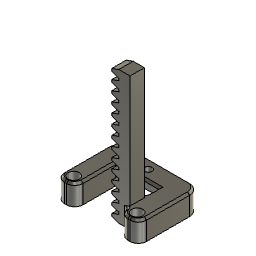
z lifter v18 (Autodesk Fusion 360 design; units mm, degrees)
Autodesk Fusion 360 part; units mm, degrees
note: some values were not read from the file. Chosen so that the rebuilt part matches the saved one: which pieces of a blend or face edit are solid.
sketch "Sketch1" plane through (0, 0, 0) normal (0, 1, 0) x (1, 0, 0)
  line L0 (20, -5) -> (-20, -5)
  line L1 (-20, -5) -> (-20, 5)
  line L2 (-20, 5) -> (20, 5)
  line L3 (20, 5) -> (20, -5)
  line L4 (20, -5) -> (-20, 5) construction
  line L5 (-20, -5) -> (20, 5) construction
  dimension "d1" = 40
  dimension "d2" = 10
  constraint horizontal L0
  constraint perpendicular L0 L1
  constraint parallel L0 L2
  constraint parallel L1 L3
  constraint coincident L4 origin
  constraint coincident L5 origin
  measures "d1" distance of L1.end L2.end
  measures "d2" distance of L0.end L1.end
extrude "Extrude1" add sketch "Sketch1" along normal blind 10 makes body 1
sketch "Sketch3" plane through (0, 0, 0) normal (0, -1, 0) x (1, 0, 0)
  line L0 (-20, -5) -> (20, -5)
  line L1 (20, -5) -> (20, 5)
  line L2 (20, 5) -> (-20, 5)
  line L3 (-20, 5) -> (-20, -5)
  line L4 (-20, 5) -> (-11, 5)
  line L5 (-11, 5) -> (-11, -5)
  line L6 (-11, -5) -> (-20, -5)
  line L7 (-20, -5) -> (-20, 5)
  line L8 (20, 5) -> (11, 5)
  line L9 (11, 5) -> (11, -5)
  line L10 (11, -5) -> (20, -5)
  line L11 (20, -5) -> (20, 5)
  dimension "d9" = 9
  dimension "d10" = 9
  constraint horizontal L4
  constraint vertical L5
  constraint horizontal L6
  constraint vertical L7
  constraint coincident L2.end L3.start
  constraint horizontal L8
  constraint vertical L9
  constraint horizontal L10
  constraint vertical L11
  constraint coincident L1.end L2.start
  measures "d9" distance of L2.end L4.end
  measures "d10" distance of L1.end L8.end
extrude "Extrude3" add sketch "Sketch3" along normal blind 20 contours L0 L2 L3 L4 L5 L6 L7 | L0 L1 L2 L8 L9 L10 L11 bodies 1
sketch "Sketch4" plane through (0, 0, 5) normal (0, 0, 1) x (-1, 0, 0)
  line L0 (-20, 20) -> (-20, -10)
  line L1 (-20, -10) -> (20, -10)
  line L2 (20, -10) -> (20, 20)
  line L3 (20, 20) -> (11, 20)
  line L4 (11, 20) -> (11, 0)
  line L5 (11, 0) -> (-11, 0)
  line L6 (-11, 0) -> (-11, 20)
  line L7 (-11, 20) -> (-20, 20)
  line L8 (-15.5, 20) -> (-15.5, 16) construction
  line L9 (15.5, 20) -> (15.5, 16) construction
  circle A0 centre (-15.5, 16) radius 2.75
  circle A1 centre (15.5, 16) radius 2.75
  dimension "d13" = 4
  dimension "d14" = 4
  dimension "d15" = 5.5
  dimension "d16" = 5.5
  constraint midpoint L7 L8.start
  constraint perpendicular L7 L8
  constraint midpoint L3 L9.start
  constraint perpendicular L3 L9
  constraint coincident L8.end A0.centre
  constraint coincident L9.end A1.centre
  measures "d13" distance of L8.start L8.end
  measures "d14" distance of L9.start L9.end
  measures "d15" diameter of A0
  measures "d16" diameter of A1
extrude "Extrude4" cut sketch "Sketch4" against normal blind 10 contours A0 | A1 bodies 1
sketch "Sketch1 (2)" plane through (0, 0, 0) normal (0, 0, 1) x (1, 0, 0) in component "Component"
  line L0 (0, 0) -> (1.2284, 3.375)
  line L1 (2.4927, 3.375) -> (3.7211, 0)
  line L2 (1.2284, 3.375) -> (2.4927, 3.375)
  line L3 (0, 0) -> (0, -5.5)
  line L4 (0, -5.5) -> (3.7211, -5.5)
  line L5 (3.7211, -5.5) -> (3.7211, 0)
  line L6 (1.6364, 0) -> (100, 0)
  line L7 (0, 0, 0) -> (0, 0, 7)
sketch "Sketch2" plane through (0, 0, 0) normal (0, 0, 1) x (1, 0, 0) in component "Component"
  line L0 (0, 0) -> (64.9821, 0)
  line L1 (0, 0) -> (0, -5.5)
  line L2 (0, -5.5) -> (64.9821, -5.5)
  line L3 (64.9821, -5.5) -> (64.9821, 0)
sweep "Sweep1" add profiles "Sketch1 (2)" path "Sketch1 (2)" along L7 section 1 separate body makes body 2 in component "Component"
pattern_path "PathPattern1" count 14 spacing 4.7124 from (1.6364, 0, 0) path "Sketch1 (2)" along L6 of "Sweep1" makes body 3 makes body 4 makes body 5 makes body 6 makes body 7 makes body 8 makes body 9 makes body 10 makes body 11 makes body 12 makes body 13 makes body 14 makes body 15 in component "Component"
extrude "Extrude1'" add sketch "Sketch2" along normal blind 7 bodies 2 3 4 5 6 7 8 9 10 11 12 13 14 15 in component "Component"
move_body "Move1" bodies 2 to x (1, 0, 0) y (0, 0, 1) z (0, -1, 0) at (0, -5.5, 5.5) in component "Component"
sketch "Sketch3 (2)" plane through (0, 0, 0) normal (0, 0, 1) x (1, 0, 0) in component "Component"
  line L0 (0, 0) -> (51.2695, 0) construction
  line L1 (51.2695, 0) -> (51.2695, 3) construction
  line L2 (51.2695, 3) -> (0, 3) construction
  line L3 (0, 3) -> (0, 0) construction
  constraint perpendicular L0 L1
  constraint parallel L0 L2
  constraint parallel L1 L3
move_body "Move2" bodies 2 to x (0, 0, 1) y (0, 1, 0) z (-1, 0, 0) at (11, -2.5, -5) in component "Component"
sketch "Sketch5" plane through (0, 0, -5) normal (0, 0, -1) x (1, 0, 0)
  circle A0 centre (-15.5, 16) radius 2.75
  circle A1 centre (15.5, 16) radius 2.75
  line L0 (-20, 20) -> (-20, -10)
  line L1 (-20, -10) -> (20, -10)
  line L2 (20, -10) -> (20, 20)
  line L3 (20, 20) -> (11, 20)
  line L4 (11, 20) -> (11, 0)
  line L5 (11, 0) -> (-11, 0)
  line L6 (-11, 0) -> (-11, 20)
  line L7 (-11, 20) -> (-20, 20)
  line L8 (-11, 0) -> (-20, 0) construction
  line L9 (11, 0) -> (20, 0) construction
  line L10 (20, -10) -> (-20, 0) construction
  line L11 (-20, -10) -> (20, 0) construction
  circle A2 centre (0, -5) radius 10.75
  circle A3 centre (0, -5) radius 1.75
  dimension "d29" = 21.5
  dimension "d32" = 3.5
  constraint coincident L5.end L6.start
  constraint coincident L0 L8.end
  constraint perpendicular L0 L8
  constraint coincident L4.end L5.start
  constraint coincident L2 L9.end
  constraint perpendicular L2 L9
  constraint coincident L1.end L2.start
  constraint coincident L0.end L1.start
  constraint midpoint L11 A2.centre
  constraint concentric A2 A3
  measures "d29" diameter of A2
  measures "d32" diameter of A3
extrude "Extrude5" cut sketch "Sketch5" against normal blind 6 contours L1 L5 A2 | A3 bodies 1
extrude "Extrude6" cut sketch "Sketch5" against normal blind 10 contours A3 bodies 1
fillet "Fillet1" radius 5 2 edges at (20, 10, 0) (-20, 10, 0) on bodies 1
fillet "Fillet2" radius 4 4 edges at (-20, -20, 0) (-11, -20, 0) (11, -20, 0) (20, -20, 0) on bodies 1
combine "Combine1" operation add target body 2 tool bodies 1 in component "Component"
fillet "Fillet1'" radius 3 2 edges at (11, -15, 0) (11, -8, 0) on bodies 2 in component "Component"
chamfer "Chamfer1" distance 1 angle 45 14 edges at (0, 0, 5) (-11, -8, 5) (-12.1716, -18.8284, 5) (-15.5, -20, 5) (-18.8284, -18.8284, 5) (-20, -5.5, 5) (-18.5355, 8.5355, 5) (0, 10, 5) (18.5355, 8.5355, 5) (20, -5.5, 5) (18.8284, -18.8284, 5) (15.5, -20, 5) (12.6095, -19.2071, 5) (10.0846, -15.5946, 5) on bodies 2 in component "Component"
sketch "Sketch6" plane through (0, 0, -5) normal (0, 0, -1) x (1, 0, 0)
  circle A0 centre (15.5, 16) radius 2.75
  arc A1 (8.2918, 15) -> (11.1667, 17.1429) centre (8.2918, 18) ccw
  line L0 (8.2918, 15) -> (5.5, 15)
  line L1 (5.5, 15) -> (5.5, 8)
  line L2 (5.5, 8) -> (8, 8)
  arc A2 (11, 5) -> (8, 8) centre (8, 5) ccw
  line L3 (11, 5) -> (11, 0)
  line L4 (11, 0) -> (9.5164, 0)
  arc A3 (9.5164, -10) -> (9.5164, 0) centre (0, -5) ccw
  line L5 (9.5164, -10) -> (15, -10)
  arc A4 (15, -10) -> (20, -5) centre (15, -5) ccw
  line L6 (20, -5) -> (20, 16)
  arc A5 (20, 16) -> (16, 20) centre (16, 16) ccw
  line L7 (16, 20) -> (15, 20)
  arc A6 (15, 20) -> (11.1667, 17.1429) centre (15, 16) ccw
  circle A7 centre (15.5, 16) radius 4.5
  constraint concentric A0 A7
  constraint coincident L6.end A7
extrude "Extrude7" [suppressed]
sketch "Sketch7" plane through (0, 0, -5) normal (0, 0, 1) x (-1, 0, 0)
  arc A0 (-20, 16) -> (-11.1006, 16.9461) centre (-15.5, 16) ccw
  arc A1 (-11.1667, 17.1429) -> (-11.1006, 16.9461) centre (-8.2918, 18) ccw
  arc A2 (-11.1667, 17.1429) -> (-15, 20) centre (-15, 16) ccw
  line L0 (-15, 20) -> (-16, 20)
  arc A3 (-16, 20) -> (-20, 16) centre (-16, 16) ccw
  circle A4 centre (-15.5, 16) radius 2.25
  dimension "d44" = 4.5
  constraint concentric A0 A4
  measures "d44" diameter of A4
extrude "Extrude8" [suppressed]
component "Component" placed x (1, 0, 0) y (0, 1, 0) z (0, 0, 1) at (0, 0, 0)
